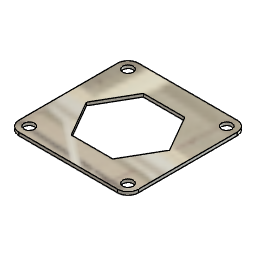
Cabeca (Autodesk Fusion 360 archive; units mm, degrees)
design "Base Cima"
Autodesk Fusion 360 part; units mm, degrees
sketch "Sketch1" plane through (0, 0, 0) normal (0, 1, 0) x (1, 0, 0)
  line L0 (47.5, -57.5) -> (-47.5, -57.5)
  line L1 (-57.5, -47.5) -> (-57.5, 47.5)
  line L2 (-47.5, 57.5) -> (47.5, 57.5)
  line L3 (57.5, 47.5) -> (57.5, -47.5)
  line L4 (57.5, -57.5) -> (-57.5, 57.5) construction
  line L5 (-57.5, -57.5) -> (57.5, 57.5) construction
  arc A0 (57.5, 47.5) -> (47.5, 57.5) centre (47.5, 47.5) ccw
  arc A1 (47.5, -57.5) -> (57.5, -47.5) centre (47.5, -47.5) ccw
  arc A2 (-57.5, -47.5) -> (-47.5, -57.5) centre (-47.5, -47.5) ccw
  arc A3 (-47.5, 57.5) -> (-57.5, 47.5) centre (-47.5, 47.5) ccw
  circle A4 centre (-47.5, 47.5) radius 5
  circle A5 centre (47.5, 47.5) radius 5
  circle A6 centre (47.5, -47.5) radius 5
  circle A7 centre (-47.5, -47.5) radius 5
  line L6 (40, 0) -> (20, 34.641)
  line L7 (20, 34.641) -> (-20, 34.641)
  line L8 (-20, 34.641) -> (-40, 0)
  line L9 (-40, 0) -> (-20, -34.641)
  line L10 (-20, -34.641) -> (20, -34.641)
  line L11 (20, -34.641) -> (40, 0)
  dimension "d1" = 115
  dimension "d2" = 115
  dimension "d3" = 10
  dimension "d4" = 10
  dimension "d5" = 10
  dimension "d6" = 10
  dimension "d7" = 10
  dimension "d8" = 10
  dimension "d9" = 40
  constraint horizontal L0
  constraint perpendicular L0 L1
  constraint parallel L0 L2
  constraint parallel L1 L3
  constraint coincident L4 origin
  constraint coincident L5 origin
  constraint coincident L5.end L2
  constraint coincident L5.end L3
  constraint tangent L2 A0
  constraint tangent L3 A0
  constraint coincident L4.start L3
  constraint coincident L4.start L0
  constraint tangent L3 A1
  constraint tangent L0 A1
  constraint equal A0 A1
  constraint coincident L5.start L0
  constraint coincident L5.start L1
  constraint tangent L0 A2
  constraint tangent L1 A2
  constraint equal A0 A2
  constraint coincident L4.end L2
  constraint coincident L4.end L1
  constraint tangent L2 A3
  constraint tangent L1 A3
  constraint concentric A3 A4
  constraint concentric A0 A5
  constraint concentric A1 A6
  constraint concentric A2 A7
  measures "d1" distance of L4.end L5.end
  measures "d2" distance of L5.start L4.end
  measures "d3" radius of A0
  measures "d4" radius of A3
  measures "d5" diameter of A4
  measures "d6" diameter of A5
  measures "d7" diameter of A6
  measures "d8" diameter of A7
  measures "d9" distance of L6.start origin
extrude "Extrude1" add sketch "Sketch1" along normal blind 3
